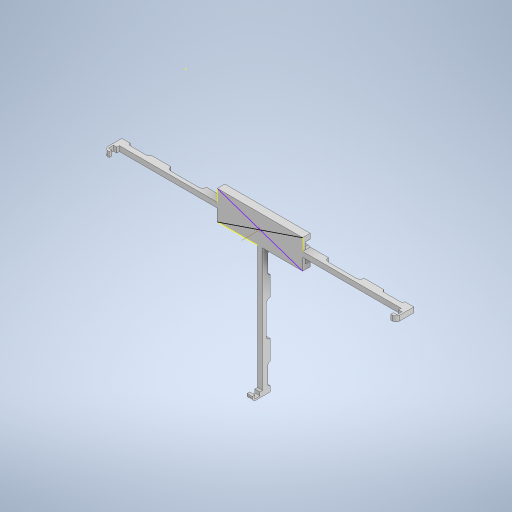
# Autodesk Inventor part: rainHolder
Saved by Autodesk Inventor 2023 (Build 270158000, 158)
## iProperties
Created: 2023-03-27
Part Number: rainHolder
Material: Générique
Document SubType Name: Modeling
Designer: eleves
Density: 1 g/cm^3
Appearance: Par défaut
Author: eleves
Autodesk Inventor part; units mm, degrees
ref_plane "YZ Plane" through (0, 0, 0) normal (1, 0, 0) x (0, 1, 0)
ref_plane "XZ Plane" through (0, 0, 0) normal (0, 1, 0) x (-1, 0, 0)
ref_plane "XY Plane" through (0, 0, 0) normal (0, 0, 1) x (1, 0, 0)
sketch "Esquisse1" plane through (0, 0, 0) normal (0, 0, 1) x (1, 0, 0)
  line L0 (-65.5174, -57.3571) -> (-65.5174, -54.3571) construction
  line L1 (-65.5174, -57.3571) -> (68.5174, -57.3571) construction
  line L2 (68.5174, -54.3571) -> (68.5174, -57.3571) construction
  line L3 (68.5174, -54.3571) -> (-65.5174, -54.3571) construction
  line L4 (-65.5174, -65.3571) -> (-65.5174, -62.3571) construction
  line L5 (-65.5174, -65.3571) -> (68.5174, -65.3571) construction
  line L6 (68.5174, -62.3571) -> (68.5174, -65.3571) construction
  line L7 (68.5174, -62.3571) -> (-65.5174, -62.3571) construction
  line L8 (68.5174, -54.3571) -> (-65.5174, -65.3571) construction
  line L9 (-65.5174, -54.3571) -> (68.5174, -65.3571) construction
  line L10 (-65.5174, -61.8571) -> (68.5174, -61.8571)
  line L11 (68.5174, -61.8571) -> (68.5174, -57.8571)
  line L12 (68.5174, -57.8571) -> (-65.5174, -57.8571)
  line L13 (-65.5174, -57.8571) -> (-65.5174, -61.8571)
  line L14 (-65.5174, -61.8571) -> (68.5174, -57.8571) construction
  line L15 (68.5174, -61.8571) -> (-65.5174, -57.8571) construction
  line L16 (68.5174, -54.3571) -> (18.5174, -54.3571)
  line L17 (18.5174, -54.3571) -> (18.5174, -51.3571)
  line L18 (18.5174, -51.3571) -> (68.5174, -51.3571)
  line L19 (68.5174, -51.3571) -> (68.5174, -54.3571)
  line L20 (68.5174, -65.3571) -> (18.5174, -65.3571)
  line L21 (18.5174, -65.3571) -> (18.5174, -68.3571)
  line L22 (18.5174, -68.3571) -> (68.5174, -68.3571)
  line L23 (68.5174, -68.3571) -> (68.5174, -65.3571)
  line L24 (18.5174, -57.8571) -> (18.5174, -61.8571)
  point P0 (0, 0)
  point P1 (1.5, -59.8571)
  dimension "d1" = 0.5
  dimension "d2" = 50
  dimension "d3" = 3
  dimension "d4" = 3
  constraints: 34 end point, 6 parallel, 4 perpendicular, 3 horizontal, 3 midpoint, 3 point on line
  measures "d1" distance between parallel lines of L1 L12
  measures "d2" distance of L17.end L18.end
  measures "d3" distance of L18.end L2.start
  measures "d4" distance of L22.end L5.end
extrude "Extrusion1" add sketch "Esquisse1" along normal blind 2.9 contours L24 L12 L11 L10 | L16 L17 L18 L19 | L23 L22 L21 L20
sketch "Esquisse2" plane through (0, 0, 2.9) normal (0, 0, 1) x (1, 0, 0)
  line L0 (68.5174, -57.8571) -> (18.5174, -57.8571) construction
  line L1 (18.5174, -61.8571) -> (68.5174, -61.8571) construction
  line L2 (68.5174, -57.8571) -> (18.5174, -61.8571) construction
  line L3 (18.5174, -57.8571) -> (18.5174, -61.8571) construction
  line L4 (18.5174, -61.8571) -> (18.5174, -57.8571) construction
  line L5 (18.5174, -57.8571) -> (18.9148, -57.8571) construction
  line L6 (18.9148, -57.8571) -> (68.5174, -61.8571) construction
  line L7 (43.7161, -59.8571) -> (126.2161, -59.8571)
  line L8 (43.7161, -59.8571) -> (-38.7839, -59.8571)
  line L9 (68.5174, -51.3571) -> (18.5174, -51.3571) projected
  line L10 (18.5174, -68.3571) -> (68.5174, -68.3571) projected
  line L11 (68.5174, -51.3571) -> (18.5174, -51.3571)
  line L12 (18.5174, -51.3571) -> (18.5174, -68.3571)
  line L13 (18.5174, -68.3571) -> (68.5174, -68.3571)
  line L14 (68.5174, -68.3571) -> (68.5174, -51.3571)
  line L15 (126.2161, -59.8571) -> (126.2161, -61.3571)
  line L16 (126.2161, -59.8571) -> (126.2161, -58.3571)
  line L17 (126.2161, -58.3571) -> (-38.7839, -58.3571)
  line L18 (-38.7839, -58.3571) -> (-38.7839, -59.8571)
  line L19 (-38.7839, -59.8571) -> (-38.7839, -61.3571)
  line L20 (-38.7839, -61.3571) -> (126.2161, -61.3571)
  point P0 (0, 0)
  point P1 (68.5174, -58.3571)
  point P2 (18.5174, -58.3571)
  point P3 (18.5174, -61.3571)
  point P4 (68.5174, -61.3571)
  dimension "d7" = 82.5
  dimension "d8" = 82.5
  dimension "d9" = 1.5
  dimension "d10" = 1.5
  constraints: 32 end point, 4 horizontal, 4 perpendicular, 3 equal length, 2 vertical, 1 midpoint, 1 point on line
  measures "d7" distance of L7.start L7.end
  measures "d8" distance of L7.start L8.end
  measures "d9" distance of L7.end L15.end
  measures "d10" distance of L7.end L16.end
extrude "Extrusion2" add sketch "Esquisse2" along normal blind 1.5
sketch "Esquisse3" plane through (0, 0, 4.4) normal (0, 0, 1) x (1, 0, 0)
  line L0 (68.5174, -51.3571) -> (18.5174, -51.3571) construction
  line L1 (18.5174, -65.3571) -> (18.5174, -68.3571) construction
  line L2 (68.5174, -51.3571) -> (18.5174, -68.3571) construction
  line L3 (18.5174, -68.3571) -> (18.5174, -51.3571) construction
  line L4 (18.5174, -68.3571) -> (68.5174, -68.3571) construction
  line L5 (68.5174, -68.3571) -> (18.5174, -51.3571) construction
  line L6 (42.0174, 20.8929) -> (45.0174, 20.8929)
  line L7 (45.0174, 20.8929) -> (45.0174, -140.6071)
  line L8 (45.0174, -140.6071) -> (42.0174, -140.6071)
  line L9 (42.0174, -140.6071) -> (42.0174, 20.8929)
  line L10 (42.0174, 20.8929) -> (45.0174, -140.6071) construction
  line L11 (45.0174, 20.8929) -> (42.0174, -140.6071) construction
  point P0 (0, 0)
  point P1 (43.5174, -59.8571)
  dimension "d13" = 3
  dimension "d14" = 161.5
  constraints: 18 end point, 3 midpoint, 2 parallel, 1 collinear, 1 horizontal, 1 perpendicular
  measures "d13" distance of L7.end L8.end
  measures "d14" distance of L8.end L6.start
extrude "Extrusion3" add sketch "Esquisse3" against normal blind 1.5
sketch "Esquisse4" plane through (0, 0, 2.9) normal (0, 0, -1) x (-1, 0, 0)
  line L0 (-45.0174, -68.3571) -> (-42.0174, -68.3571) projected
  line L1 (-45.0174, -68.3571) -> (-45.0174, -140.6071) projected
  line L2 (-45.0174, -140.6071) -> (-42.0174, -140.6071) projected
  line L3 (-42.0174, -140.6071) -> (-42.0174, -68.3571) projected
  line L4 (-68.5174, -61.3571) -> (-68.5174, -58.3571) projected
  line L5 (-126.2161, -58.3571) -> (-68.5174, -58.3571) projected
  line L6 (-126.2161, -61.3571) -> (-126.2161, -58.3571) projected
  line L7 (-68.5174, -61.3571) -> (-126.2161, -61.3571) projected
  line L8 (-18.5174, -58.3571) -> (-18.5174, -61.3571) projected
  line L9 (38.7839, -61.3571) -> (-18.5174, -61.3571) projected
  line L10 (38.7839, -58.3571) -> (38.7839, -61.3571) projected
  line L11 (-18.5174, -58.3571) -> (38.7839, -58.3571) projected
  line L12 (-42.0174, -51.3571) -> (-45.0174, -51.3571) projected
  line L13 (-42.0174, -51.3571) -> (-42.0174, 20.8929) projected
  line L14 (-42.0174, 20.8929) -> (-45.0174, 20.8929) projected
  line L15 (-45.0174, 20.8929) -> (-45.0174, -51.3571) projected
  point P0 (0, 0)
extrude "Extrusion4" add sketch "Esquisse4" along normal up to surface (2.9 mm away)
sketch "Esquisse5" plane through (0, 0, 4.4) normal (0, 0, 1) x (1, 0, 0)
  line L0 (126.2161, -58.3571) -> (126.2161, -61.3571) projected
  line L1 (126.2161, -58.3571) -> (129.2161, -58.3571)
  line L2 (129.2161, -58.3571) -> (129.2161, -61.3571)
  line L3 (129.2161, -61.3571) -> (126.2161, -61.3571)
  line L4 (126.2161, -61.3571) -> (126.2161, -58.3571)
  line L5 (42.0174, 20.8929) -> (45.0174, 20.8929)
  line L6 (45.0174, 20.8929) -> (45.0174, 23.8929)
  line L7 (45.0174, 23.8929) -> (42.0174, 23.8929)
  line L8 (42.0174, 23.8929) -> (42.0174, 20.8929)
  line L9 (45.0174, -68.3571) -> (68.5174, -68.3571) projected
  line L10 (68.5174, -68.3571) -> (68.5174, -61.3571) projected
  line L11 (68.5174, -61.3571) -> (126.2161, -61.3571) projected
  line L12 (126.2161, -61.3571) -> (126.2161, -58.3571) projected
  line L13 (126.2161, -58.3571) -> (68.5174, -58.3571) projected
  line L14 (68.5174, -58.3571) -> (68.5174, -51.3571) projected
  line L15 (68.5174, -51.3571) -> (45.0174, -51.3571) projected
  line L16 (45.0174, -51.3571) -> (45.0174, 20.8929) projected
  line L17 (45.0174, 20.8929) -> (42.0174, 20.8929) projected
  line L18 (42.0174, 20.8929) -> (42.0174, -51.3571) projected
  line L19 (42.0174, -51.3571) -> (18.5174, -51.3571) projected
  line L20 (18.5174, -51.3571) -> (18.5174, -58.3571) projected
  line L21 (18.5174, -58.3571) -> (-38.7839, -58.3571) projected
  line L22 (-38.7839, -58.3571) -> (-38.7839, -61.3571) projected
  line L23 (-38.7839, -61.3571) -> (18.5174, -61.3571) projected
  line L24 (18.5174, -61.3571) -> (18.5174, -68.3571) projected
  line L25 (18.5174, -68.3571) -> (42.0174, -68.3571) projected
  line L26 (42.0174, -68.3571) -> (42.0174, -140.6071) projected
  line L27 (42.0174, -140.6071) -> (45.0174, -140.6071) projected
  line L28 (45.0174, -140.6071) -> (45.0174, -68.3571) projected
  line L29 (45.0174, -140.6071) -> (42.0174, -140.6071)
  line L30 (42.0174, -140.6071) -> (42.0174, -143.6071)
  line L31 (42.0174, -143.6071) -> (45.0174, -143.6071)
  line L32 (45.0174, -143.6071) -> (45.0174, -140.6071)
  line L33 (-38.7839, -58.3571) -> (-41.7839, -58.3571)
  line L34 (-41.7839, -58.3571) -> (-41.7839, -61.3571)
  line L35 (-41.7839, -61.3571) -> (-38.7839, -61.3571)
  line L36 (-38.7839, -61.3571) -> (-38.7839, -58.3571)
  point P0 (0, 0)
  dimension "d19" = 3
  dimension "d20" = 3
  dimension "d21" = 3
  dimension "d22" = 3
  constraints: 32 end point, 8 parallel, 4 horizontal, 4 perpendicular, 2 collinear
  measures "d19" distance of L0.start L1.end
  measures "d20" distance of L7.end L5.start
  measures "d21" distance of L31.end L27.end
  measures "d22" distance of L34.end L35.end
sketch "Esquisse6" plane through (0, 0, 4.4) normal (0, 0, 1) x (1, 0, 0)
  line L0 (42.0174, -51.3571) -> (18.5174, -51.3571) projected
  line L1 (51.8024, 29.9125) -> (32.5484, 29.9125)
  line L2 (32.5484, 29.9125) -> (32.5484, -51.3571)
  line L3 (32.5484, -51.3571) -> (51.8024, -51.3571)
  line L4 (51.8024, -51.3571) -> (51.8024, 29.9125)
  point P0 (0, 0)
  constraints: 8 end point, 2 parallel, 1 horizontal, 1 perpendicular, 1 point on line
extrude "Extrusion5" cut sketch "Esquisse6" against normal blind 10
extrude "Extrusion6" add sketch "Esquisse5" along normal blind 6 and the other way blind 4.4 contours L1 L2 L3 L0 | L32 L31 L30 L27 | L22 L35 L34 L33
sketch "Esquisse7" plane through (126.2161, -61.3571, 4.4) normal (-1, 0, 0) x (0, 0, 1)
  line L0 (0, 3) -> (6, 3) projected
  line L1 (0, 0) -> (6, 0) projected
  line L2 (4.5, 3) -> (1.5, 3)
  line L3 (1.5, 3) -> (1.5, 0)
  line L4 (1.5, 0) -> (4.5, 0)
  line L5 (4.5, 0) -> (4.5, 3)
  line L6 (6, 3) -> (6, 0) projected
  point P0 (-4.4, 61.3571)
  point P1 (4.5, 0)
  dimension "d29" = 3
  dimension "d30" = 1.5
  constraints: 8 end point, 2 parallel, 2 point on line, 1 horizontal, 1 perpendicular
  measures "d29" distance between parallel lines of L5 L3
  measures "d30" distance between parallel lines of L6 L5
extrude "Extrusion7" cut sketch "Esquisse7" against normal blind 2 contours L0 L5 L1 L3
sketch "Esquisse8" plane through (-38.7839, -61.3571, 4.4) normal (1, 0, 0) x (0, 0, -1)
  line L0 (-1.5, 3) -> (-4.5, 3) projected
  line L1 (-1.5, 0) -> (-1.5, 3) projected
  line L2 (-4.5, 0) -> (-1.5, 0) projected
  line L3 (-4.5, 3) -> (-4.5, 0) projected
  point P0 (4.4, 61.3571)
extrude "Extrusion8" cut sketch "Esquisse8" against normal blind 2
sketch "Esquisse9" plane through (42.0174, -140.6071, 4.4) normal (0, 1, 0) x (1, 0, 0)
  line L0 (3, 4.4) -> (3, -6) projected
  line L1 (0, -6) -> (0, 4.4) projected
  line L2 (3, -4.5) -> (0, -4.5)
  line L3 (0, -4.5) -> (0, -1.5)
  line L4 (0, -1.5) -> (3, -1.5)
  line L5 (3, -1.5) -> (3, -4.5)
  line L6 (3, -6) -> (0, -6) projected
  point P0 (-42.0174, 4.4)
  point P1 (3, -1.5)
  point P2 (0, -4.5)
  dimension "d35" = 3
  dimension "d36" = 1.5
  constraints: 8 end point, 2 parallel, 2 point on line, 1 horizontal, 1 perpendicular
  measures "d35" distance between parallel lines of L4 L2
  measures "d36" distance between parallel lines of L6 L2
extrude "Extrusion9" cut sketch "Esquisse9" against normal blind 2 contours L0 L2 L1 L4
fillet "Congé1" radius 2 3 edges at (43.5174, -143.6071, 10.4) (129.2161, -59.8571, 10.4) (-41.7839, -59.8571, 10.4)
sketch "Esquisse10" plane through (45.0174, -68.3571, 4.4) normal (1, 0, 0) x (0, 0, -1)
  line L0 (4.4, 0) -> (4.4, -75.25) construction
  line L1 (4.4, -75.25) -> (4.4, 0) construction
  line L2 (4.4, 0) -> (4.4, -37.625) construction
  line L3 (4.4, 0) -> (4.4, -37.625) construction
  line L4 (4.4, -37.625) -> (4.4, -75.25) construction
  line L5 (4.4, -45.7726) -> (4.4, -29.4774) construction
  line L6 (6.7186, -45.7726) -> (6.7186, -29.4774)
  line L7 (2.0814, -29.4774) -> (2.0814, -45.7726)
  arc A0 (2.0814, -45.7726) -> (6.7186, -45.7726) centre (4.4, -45.7726) ccw
  arc A1 (6.7186, -29.4774) -> (2.0814, -29.4774) centre (4.4, -29.4774) ccw
  line L8 (4.4, -18.8125) -> (4.4, 0)
  line L9 (4.4, -56.4375) -> (4.4, -75.25)
  line L10 (4.4, -70.7239) -> (4.4, -60.9636) construction
  line L11 (5.7039, -70.7239) -> (5.7039, -60.9636)
  line L12 (3.0961, -60.9636) -> (3.0961, -70.7239)
  arc A2 (3.0961, -70.7239) -> (5.7039, -70.7239) centre (4.4, -70.7239) ccw
  arc A3 (5.7039, -60.9636) -> (3.0961, -60.9636) centre (4.4, -60.9636) ccw
  line L13 (4.4, -14.2864) -> (4.4, -4.5261) construction
  line L14 (5.7039, -14.2864) -> (5.7039, -4.5261)
  line L15 (3.0961, -4.5261) -> (3.0961, -14.2864)
  arc A4 (3.0961, -14.2864) -> (5.7039, -14.2864) centre (4.4, -14.2864) ccw
  arc A5 (5.7039, -4.5261) -> (3.0961, -4.5261) centre (4.4, -4.5261) ccw
  point P0 (4.4, 68.3571)
  point P1 (4.4, -65.8438)
  point P2 (4.4, -9.4063)
  constraints: 36 end point, 12 point on circle, 12 tangent, 8 midpoint, 6 centre point, 5 collinear, 3 parallel, 3 point on line, 1 vertical
extrude "Extrusion10" cut sketch "Esquisse10" against normal blind 6
sketch "Esquisse11" plane through (0, 0, 4.4) normal (0, 0, 1) x (1, 0, 0)
  line L0 (68.5174, -58.3571) -> (68.5174, -51.3571) projected
  line L1 (18.5174, -68.3571) -> (42.0174, -68.3571) projected
  line L2 (68.5174, -51.3571) -> (18.5174, -68.3571)
  line L3 (18.5174, -51.3571) -> (18.5174, -58.3571) projected
  line L4 (18.5174, -51.3571) -> (68.5174, -68.3571)
  point P0 (0, 0)
  point P1 (43.5174, -59.8571)
  constraints: 4 end point, 1 midpoint
pattern_circular "Réseau circulaire1" count 4 over 360 about axis through (43.5174, -59.8571, 4.4) along (0, 0, 1) of "Extrusion10"
sketch "Esquisse12" plane through (18.5174, -61.8571, 2.9) normal (0, -1, 0) x (1, 0, 0)
  line L0 (49.0903, -2.9) -> (36.7222, -2.9) projected
  arc A0 (49.0903, -2.9) -> (47.7864, -1.5961) centre (47.7864, -2.9) ccw projected
  line L1 (38.0261, -1.5961) -> (47.7864, -1.5961) projected
  arc A1 (38.0261, -1.5961) -> (36.7222, -2.9) centre (38.0261, -2.9) ccw projected
  line L2 (0.9097, -2.9) -> (13.2778, -2.9) projected
  arc A2 (2.2136, -1.5961) -> (0.9097, -2.9) centre (2.2136, -2.9) ccw projected
  line L3 (11.9739, -1.5961) -> (2.2136, -1.5961) projected
  arc A3 (13.2778, -2.9) -> (11.9739, -1.5961) centre (11.9739, -2.9) ccw projected
  point P0 (-18.5174, -2.9)
extrude "Extrusion11" add sketch "Esquisse12" against normal up to surface (4 mm away)
fillet "Congé2" radius 2 4 edges at (18.5174, -61.8571, 1.45) (18.5174, -57.8571, 1.45) (68.5174, -57.8571, 1.45) (68.5174, -61.8571, 1.45)
